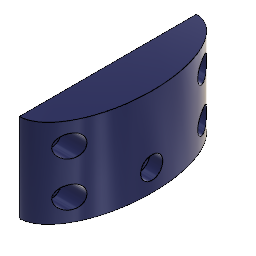
2-4080_c-beam_endcap_V5 v2 (Autodesk Fusion 360 design; units mm, degrees)
Autodesk Fusion 360 part; units mm, degrees
note: some values were not read from the file. Set by a fixed rule: which sketch regions a step uses.
sketch "MainProfile" plane through (0, 0, 0) normal (0, 0, 1) x (1, 0, 0)
  ellipse E0 centre (0, 0) end of major axis (0, -40) minor radius 20
  line L0 (0, 40) -> (0, -40)
  line L1 (-20, 0) -> (20, 0)
  dimension "d1" = 80
  dimension "d2" = 40
  constraint coincident E0.centre origin
  constraint vertical L0
  constraint coincident E0 L0.start
  constraint coincident E0 L0.end
  constraint coincident E0 L1.start
  constraint coincident E0 L1.end
  measures "d1" distance of E0
  measures "d2" distance of E0
extrude "Extrude1" add sketch "MainProfile" along normal blind 40 contours E0 L0 L1 | E0 L0 L1 picked at (4.4716, -23.2225) picked at (4.1785, 23.7227)
sketch "Holes" plane through (0, 0, 0) normal (1, 0, 0) x (0, 1, 0)
  circle A0 centre (0, 10) radius 5
  circle A1 centre (0, 10) radius 2.75
  circle A2 centre (-30, 10) radius 2.75
  circle A3 centre (-30, 10) radius 5
  circle A4 centre (30, 10) radius 2.75
  circle A5 centre (30, 10) radius 5
  circle A6 centre (-30, 30) radius 2.75
  circle A7 centre (-30, 30) radius 5
  circle A8 centre (30, 30) radius 2.75
  circle A9 centre (30, 30) radius 5
  dimension "d5" = 10
  dimension "d6" = 5.5
  dimension "d9" = 30
  dimension "d10" = 20
  dimension "d11" = 10
  constraint concentric A0 A1
  constraint vertical origin A0.centre
  measures "d5" diameter of A0
  measures "d6" diameter of A1
  measures "d11" distance of origin A0.centre
extrude "Extrude2" cut sketch "Holes" along normal blind 50 contours A1 | A2 | A4 | A6 | A8
extrude "Extrude3" cut sketch "Holes" along normal blind 30 from surface at 14 contours A0
extrude "Extrude4" cut sketch "Holes" along normal blind 30 from surface at 4.5 contours A3 | A5 | A7 | A9
sketch "Back Features" plane through (0, 0, 0) normal (-1, 0, 0) x (0, -1, 0)
  circle A0 centre (0, 10) radius 2.75
  circle A1 centre (30, 30) radius 2.75
  circle A2 centre (-30, 10) radius 2.75
  circle A3 centre (30, 10) radius 2.75
  circle A4 centre (-30, 30) radius 2.75
  line L0 (-40, 0) -> (40, 0)
  line L1 (40, 0) -> (40, 40)
  line L2 (40, 40) -> (-40, 40)
  line L3 (-40, 40) -> (-40, 0)
  line L4 (0, 40) -> (0, 0) construction
  line L5 (37.9541, 21.6763) -> (37.9541, 18.2294)
  line L6 (37.9541, 18.2294) -> (36.9391, 18.2294)
  line L7 (36.9391, 18.2294) -> (32.7752, 14.1022)
  line L8 (32.7752, 14.1022) -> (27.2498, 14.1022)
  line L9 (27.2498, 14.1022) -> (23.0858, 18.2294)
  line L10 (23.0858, 18.2294) -> (22.062, 18.2294)
  line L11 (22.062, 18.2294) -> (22.062, 20.6562)
  line L12 (22.062, 20.6562) -> (27.2542, 25.7948)
  line L13 (27.2542, 25.7948) -> (32.7743, 25.7948)
  line L14 (32.7743, 25.7948) -> (36.9231, 21.6821)
  line L15 (36.9231, 21.6821) -> (37.9541, 21.6763)
  line L16 (40, 40) -> (0, 0) construction
  line L17 (20.6562, 22.062) -> (25.7948, 27.2542)
  line L18 (25.7948, 27.2542) -> (25.7948, 32.7743)
  line L19 (25.7948, 32.7743) -> (21.6821, 36.9231)
  line L20 (21.6821, 36.9231) -> (21.6763, 37.9541)
  line L21 (21.6763, 37.9541) -> (18.2294, 37.9541)
  line L22 (18.2294, 37.9541) -> (18.2294, 36.9391)
  line L23 (18.2294, 36.9391) -> (14.1022, 32.7752)
  line L24 (14.1022, 32.7752) -> (14.1022, 27.2498)
  line L25 (14.1022, 27.2498) -> (18.2294, 23.0858)
  line L26 (18.2294, 23.0858) -> (18.2294, 22.062)
  line L27 (18.2294, 22.062) -> (20.6562, 22.062)
  line L28 (-36.9391, 18.2294) -> (-32.7752, 14.1022)
  line L29 (-32.7752, 14.1022) -> (-27.2498, 14.1022)
  line L30 (-14.1022, 27.2498) -> (-18.2294, 23.0858)
  line L31 (-18.2294, 37.9541) -> (-18.2294, 36.9391)
  line L32 (-27.2498, 14.1022) -> (-23.0858, 18.2294)
  line L33 (-18.2294, 36.9391) -> (-14.1022, 32.7752)
  line L34 (-36.9231, 21.6821) -> (-37.9541, 21.6763)
  line L35 (-25.7948, 27.2542) -> (-25.7948, 32.7743)
  line L36 (-18.2294, 23.0858) -> (-18.2294, 22.062)
  line L37 (-14.1022, 32.7752) -> (-14.1022, 27.2498)
  line L38 (-20.6562, 22.062) -> (-25.7948, 27.2542)
  line L39 (-22.062, 18.2294) -> (-22.062, 20.6562)
  line L40 (-37.9541, 18.2294) -> (-36.9391, 18.2294)
  line L41 (-37.9541, 21.6763) -> (-37.9541, 18.2294)
  line L42 (-23.0858, 18.2294) -> (-22.062, 18.2294)
  line L43 (-27.2542, 25.7948) -> (-32.7743, 25.7948)
  line L44 (-25.7948, 32.7743) -> (-21.6821, 36.9231)
  line L45 (-21.6821, 36.9231) -> (-21.6763, 37.9541)
  line L46 (-22.062, 20.6562) -> (-27.2542, 25.7948)
  line L47 (-18.2294, 22.062) -> (-20.6562, 22.062)
  line L48 (-21.6763, 37.9541) -> (-18.2294, 37.9541)
  line L49 (-32.7743, 25.7948) -> (-36.9231, 21.6821)
  line L50 (-1.7126, 37.8971) -> (1.7326, 37.8971)
  line L51 (1.7326, 37.8971) -> (1.7326, 36.8845)
  line L52 (1.7326, 36.8845) -> (5.8595, 32.6983)
  line L53 (5.8595, 32.6983) -> (5.8595, 27.1977)
  line L54 (5.8595, 27.1977) -> (1.7326, 23.0284)
  line L55 (1.7326, 23.0284) -> (1.7326, 22.0075)
  line L56 (1.7326, 22.0075) -> (-1.7156, 22.0075)
  line L57 (-1.7156, 22.0075) -> (-1.7156, 23.0253)
  line L58 (-1.7156, 23.0253) -> (-5.8413, 27.2055)
  line L59 (-5.8413, 27.2055) -> (-5.8413, 32.7023)
  line L60 (-5.8413, 32.7023) -> (-1.7156, 36.8813)
  line L61 (-1.7156, 36.8813) -> (-1.7126, 37.8971)
  constraint midpoint L2 L4.start
  constraint coincident L4.end L16.end
  constraint perpendicular L2 L5
  constraint perpendicular L5 L6
  constraint parallel L2 L8
  constraint parallel L2 L10
  constraint perpendicular L2 L11
  constraint parallel L2 L13
  constraint coincident L1.end L2.start
  constraint symmetric L5.start L16 L20.end
  constraint symmetric L5.end L16 L21.end
  constraint symmetric L6.end L16 L22.end
  constraint symmetric L7.end L16 L23.end
  constraint symmetric L8.end L16 L24.end
  constraint symmetric L9.end L16 L25.end
  constraint symmetric L10.end L16 L26.end
  constraint symmetric L11.end L16 L17.start
  constraint symmetric L12.end L16 L17.end
  constraint symmetric L13.end L16 L18.end
  constraint symmetric L14.end L16 L19.end
  constraint symmetric L4 L5.start L34.end
  constraint symmetric L4 L5.end L40.start
  constraint symmetric L4 L6.end L28.start
  constraint symmetric L4 L7.end L28.end
  constraint symmetric L4 L8.end L29.end
  constraint symmetric L4 L9.end L32.end
  constraint symmetric L4 L10.end L39.start
  constraint symmetric L4 L11.end L39.end
  constraint symmetric L4 L12.end L43.start
  constraint symmetric L4 L13.end L43.end
  constraint symmetric L4 L14.end L34.start
  constraint symmetric L4 L17.start L38.start
  constraint symmetric L4 L17.end L35.start
  constraint symmetric L4 L18.end L35.end
  constraint symmetric L4 L19.end L44.end
  constraint symmetric L4 L20.end L45.end
  constraint symmetric L4 L21.end L31.start
  constraint symmetric L4 L22.end L31.end
  constraint symmetric L4 L23.end L33.end
  constraint symmetric L4 L24.end L30.start
  constraint symmetric L4 L25.end L30.end
  constraint symmetric L4 L26.end L36.end
  constraint parallel L2 L50
  constraint perpendicular L2 L51
  constraint perpendicular L2 L53
  constraint perpendicular L2 L55
  constraint perpendicular L55 L56
  constraint perpendicular L2 L57
  constraint perpendicular L2 L59
extrude "Extrude5" add sketch "Back Features" along normal blind 1.75 contours L5 L6 L7 L8 L9 L10 L11 L12 L13 L14 L15 | L17 L18 L19 L20 L21 L22 L23 L24 L25 L26 L27 | L28 L29 L32 L34 L39 L40 L41 L42 L43 L46 L49 | L30 L31 L33 L35 L36 L37 L38 L44 L45 L47 L48 | L50 L51 L52 L53 L54 L55 L56 L57 L58 L59 L60 L61
named bodies: "2-4080 c-beam endcap"
